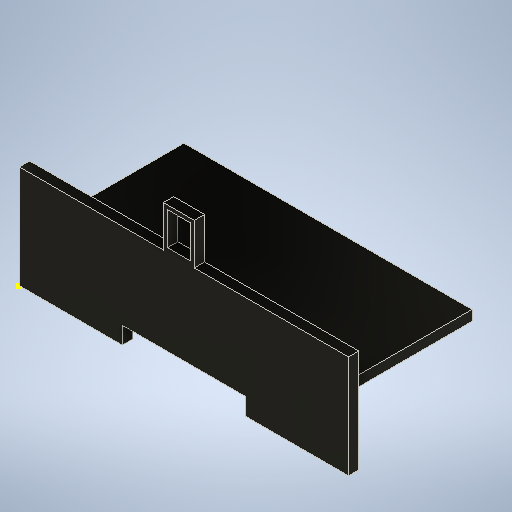
# Autodesk Inventor part: COVER_1
Saved by Autodesk Inventor 2025.3 (Build 293356030, 356C)
## iProperties
Created: 2026-06-30
Part Number: COVER_1
Material: ABS Plastic
Document SubType Name: Modeling
Designer: user
Density: 1.06 g/cm^3
Appearance: Gunmetal
Author: user
Autodesk Inventor part; units mm, degrees
ref_plane "YZ Plane" through (0, 0, 0) normal (1, 0, 0) x (0, 1, 0)
ref_plane "XZ Plane" through (0, 0, 0) normal (0, 1, 0) x (-1, 0, 0)
ref_plane "XY Plane" through (0, 0, 0) normal (0, 0, 1) x (1, 0, 0)
sketch "Sketch1" plane through (0, 0, 0) normal (0, 0, 1) x (1, 0, 0)
  line L0 (0, 0) -> (160, 0)
  line L1 (160, 0) -> (160, 50)
  line L2 (160, 50) -> (0, 50)
  line L3 (0, 50) -> (0, 0)
  line L4 (50, 0) -> (110, 0)
  line L5 (110, 0) -> (110, 8.3313)
  line L6 (110, 8.3313) -> (50, 8.3313)
  line L7 (50, 8.3313) -> (50, 0)
  line L8 (0, 50) -> (160, 50)
  line L9 (160, 50) -> (160, 45)
  line L10 (0, 45) -> (0, 50)
  line L11 (150, 50) -> (10, 50)
  line L12 (10, 30) -> (150, 30)
  line L13 (150, 30) -> (150, 25)
  line L14 (150, 25) -> (10, 25)
  line L15 (10, 25) -> (10, 30)
  dimension "d0" = 160
  dimension "d1" = 50
  dimension "d2" = 60
  dimension "d3" = 50
  dimension "d11" = 140
  dimension "d12" = 10
  dimension "d13" = 20
  dimension "d14" = 5
  constraints: 32 end point, 7 parallel, 5 horizontal, 4 perpendicular, 3 point on line
  measures "d0" distance of L2.end L1.end
  measures "d1" distance of L0.end L1.end
  measures "d2" distance of L6.end L5.end
  measures "d3" distance between parallel lines of L1 L5
  measures "d11" distance of L13.end L14.end
  measures "d12" distance between parallel lines of L3 L15
  measures "d13" distance between parallel lines of L2 L12
  measures "d14" distance between parallel lines of L14 L12
extrude "Extrusion1" add sketch "Sketch1" along normal blind 5 contours L3 L2 L1 L0 L5 L6 L7 | L12 L13 L14 L15
extrude "Extrusion2" add sketch "Sketch1" against normal blind 65 contours L12 L13 L14 L15
sketch "Sketch2" plane through (0, 0, 5) normal (0, 0, 1) x (1, 0, 0)
  line L0 (160, 50) -> (0, 50) projected
  line L1 (70, 50) -> (85, 50)
  line L2 (85, 50) -> (85, 70)
  line L3 (85, 70) -> (70, 70)
  line L4 (70, 70) -> (70, 50)
  line L5 (72, 68) -> (83, 68)
  line L6 (83, 68) -> (83, 52)
  line L7 (83, 52) -> (72, 52)
  line L8 (72, 52) -> (72, 68)
  point P0 (0, 0)
  dimension "d15" = 15
  dimension "d16" = 20
  dimension "d17" = 2
  constraints: 16 end point, 4 parallel, 2 perpendicular, 1 horizontal, 1 point on line, 3 other
  measures "d15" distance of L3.end L2.end
  measures "d16" distance of L2.end L1.end
  measures "d17" distance between parallel lines of L3 L5
extrude "Extrusion3" add sketch "Sketch2" against normal blind 5
sketch "Sketch3" plane through (0, 0, 5) normal (0, 0, 1) x (1, 0, 0)
  point P0 (0, 0)
body "Solid1"
